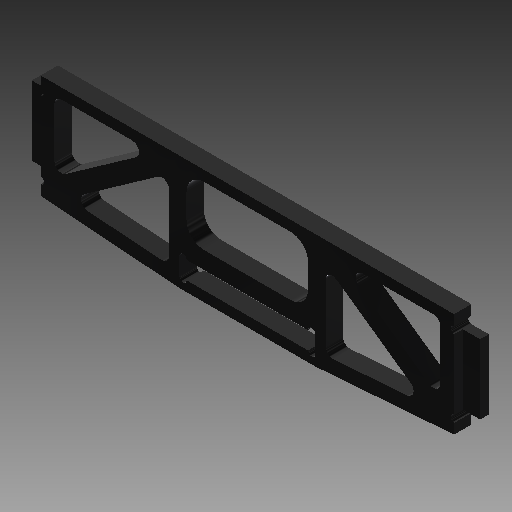
# Autodesk Inventor part: コックピット_サブフレーム_1_6
Saved by Autodesk Inventor 2018 (Build 220112000, 112)
## iProperties
Category: コックピット
Created: 2016-05-09
Part Number: コックピット_サブフレーム_1_6
Material: アセタール樹脂、黒
Document SubType Name: Modeling
Designer: hiroaki
Density: 1.425 g/cm^3
Appearance: 滑らか - 黒
Mass: 13.7144 g
Surface Area: 80.4855 cm^2
Volume: 9.62414 cm^3
Author: hiroaki
Autodesk Inventor part; units mm, degrees
ref_plane "YZ Plane" through (0, 0, 0) normal (1, 0, 0) x (0, 1, 0)
ref_plane "XZ Plane" through (0, 0, 0) normal (0, 1, 0) x (-1, 0, 0)
ref_plane "XY Plane" through (0, 0, 0) normal (0, 0, 1) x (1, 0, 0)
sketch "スケッチ1" plane through (0, 0, 0) normal (0, 0, 1) x (1, 0, 0)
  line L0 (-59.5, -15) -> (59.5, -15) construction
  line L1 (59.5, -15) -> (59.5, 15) construction
  line L2 (59.5, 15) -> (-59.5, 15) construction
  line L3 (-59.5, 15) -> (-59.5, -15) construction
  line L4 (-59.5, -15) -> (59.5, 15) construction
  line L5 (59.5, -15) -> (-59.5, 15) construction
  line L6 (-59.5, 12.1) -> (-59.5, 15)
  line L7 (-59.5, 15) -> (59.5, 15)
  line L8 (59.5, 15) -> (59.5, 12.1)
  line L9 (-59.5, -12.1) -> (-59.5, -15)
  line L10 (59.5, -15) -> (59.5, -12.1)
  line L11 (-59.5, 10) -> (-64.5, 10)
  line L12 (-64.5, 10) -> (-64.5, -10)
  line L13 (-64.5, -10) -> (-59.5, -10)
  arc A0 (-59.5, 10) -> (-59.5, 12.1) centre (-59.5, 11.05) ccw
  line L14 (0, 0) -> (0, 15) construction
  line L15 (0, 0) -> (-59.5, 0) construction
  arc A1 (-59.5, -12.1) -> (-59.5, -10) centre (-59.5, -11.05) ccw
  line L16 (59.5, 10) -> (64.5, 10)
  line L17 (64.5, 10) -> (64.5, -10)
  line L18 (64.5, -10) -> (59.5, -10)
  arc A2 (59.5, 12.1) -> (59.5, 10) centre (59.5, 11.05) ccw
  arc A3 (59.5, -10) -> (59.5, -12.1) centre (59.5, -11.05) ccw
  line L19 (-59.5, -15) -> (-19.5, -18)
  line L20 (-19.5, -18) -> (19.5, -18)
  line L21 (19.5, -18) -> (59.5, -15)
  line L22 (-19.5, -10) -> (19.5, -10) construction
  line L23 (19.5, -10) -> (19.5, -15) construction
  line L24 (19.5, -15) -> (-19.5, -15) construction
  line L25 (-19.5, -15) -> (-19.5, -10) construction
  line L26 (19.55, -9.95) -> (-19.55, -9.95)
  line L27 (-19.55, -9.95) -> (-19.55, -15.05)
  line L28 (-19.55, -15.05) -> (19.55, -15.05)
  line L29 (19.55, -15.05) -> (19.55, -9.95)
  circle A4 centre (-18.5, -9.95) radius 1.05
  circle A5 centre (-18.5, -15.05) radius 1.05
  circle A6 centre (18.5, -9.95) radius 1.05
  circle A7 centre (18.5, -15.05) radius 1.05
  dimension "d9" = 2.1
  dimension "d0" = 119
  dimension "d1" = 30
  dimension "d2" = 1.05
  dimension "d3" = 20
  dimension "d4" = 5
  dimension "d5" = 5
  dimension "d6" = 0.05
  dimension "d7" = 39
  dimension "d8" = 3
  constraints: 60 end point, 9 perpendicular, 8 point on circle, 6 collinear, 6 parallel, 6 vertical alignment, 5 horizontal, 4 centre point, 4 horizontal alignment, 4 midpoint, 4 point on line, 4 tangent, 3 equal radius, 2 symmetric about line, 2 vertical, 15 other
  measures "d0" distance of L1.end L2.end
  measures "d1" distance of L0.end L1.end
  measures "d2" radius of A0
  measures "d3" distance of L11.end L12.end
  measures "d4" distance between parallel lines of L3 L12
  measures "d5" distance of L24.end L22.start
  measures "d6" distance between parallel lines of L26 L22
  measures "d7" distance of L22.start L22.end
  measures "d8" distance between parallel lines of L20 L0
extrude "押し出し1" add sketch "スケッチ1" along normal blind 5
sketch "スケッチ2" plane through (0, 0, 5) normal (0, 0, 1) x (1, 0, 0)
  line L0 (59.5, 12.1) -> (59.5, 15) projected
  line L1 (-59.5, 15) -> (-59.5, 12.1) projected
  line L2 (65.6261, 13.972) -> (59.5, 13.972)
  line L3 (59.5, 13.972) -> (59.5, -16.1)
  line L4 (59.5, -16.1) -> (65.6261, -16.1)
  line L5 (65.6261, -16.1) -> (65.6261, 13.972)
  line L6 (-65.8886, -16.1) -> (-59.5, -16.1)
  line L7 (-59.5, -16.1) -> (-59.5, 18.3327)
  line L8 (-59.5, 18.3327) -> (-65.8886, 18.3327)
  line L9 (-65.8886, 18.3327) -> (-65.8886, -16.1)
  point P0 (0, 0)
  constraints: 16 end point, 4 parallel, 2 collinear, 2 horizontal, 2 perpendicular, 1 point on line
extrude "押し出し2" cut sketch "スケッチ2" against normal blind 2.5
sketch "スケッチ8" plane through (0, 0, 5) normal (0, 0, 1) x (1, 0, 0)
  line L0 (59.5, 15) -> (-59.5, 15) projected
  line L1 (-59.5, 10) -> (-59.5, -10) projected
  line L2 (-59.5, -15) -> (-19.5, -18) projected
  line L3 (17.45, -15.05) -> (-17.45, -15.05) projected
  arc A0 (-19.55, -15.05) -> (-17.45, -15.05) centre (-18.5, -15.05) ccw projected
  line L4 (-19.55, -15.05) -> (-19.55, -9.95) projected
  arc A1 (-17.45, -9.95) -> (-19.55, -9.95) centre (-18.5, -9.95) ccw projected
  line L5 (-17.45, -9.95) -> (17.45, -9.95) projected
  arc A2 (19.55, -9.95) -> (17.45, -9.95) centre (18.5, -9.95) ccw projected
  line L6 (19.55, -9.95) -> (19.55, -15.05) projected
  arc A3 (17.45, -15.05) -> (19.55, -15.05) centre (18.5, -15.05) ccw projected
  line L7 (-55.5, 12) -> (-22.5, 12) construction
  line L8 (-22.5, 12) -> (-22.5, -13.7638) construction
  line L9 (-22.5, -13.7638) -> (-55.5, -11.2888) construction
  line L10 (-55.5, -11.2888) -> (-55.5, 12) construction
  line L11 (17.5013, -10) -> (-17.5013, -10) construction
  arc A4 (-17.5013, -10) -> (-19.5, -9.95) centre (-18.5, -9.95) ccw construction
  line L12 (-19.5, -9.95) -> (-19.5, -15.05) construction
  arc A5 (-19.5, -15.05) -> (-17.5013, -15) centre (-18.5, -15.05) ccw construction
  line L13 (-17.5013, -15) -> (17.5013, -15) construction
  arc A6 (17.5013, -15) -> (19.5, -15.05) centre (18.5, -15.05) ccw construction
  line L14 (19.5, -15.05) -> (19.5, -9.95) construction
  arc A7 (19.5, -9.95) -> (17.5013, -10) centre (18.5, -9.95) ccw construction
  line L15 (-17.5, 12) -> (17.5, 12)
  line L16 (17.5, 12) -> (17.5, -5)
  line L17 (17.5, -5) -> (-17.5, -5)
  line L18 (-17.5, -5) -> (-17.5, 12)
  line L19 (0, 0) -> (0, 15) construction
  line L20 (-22.5, 12) -> (-55.5, -11.2888) construction
  line L21 (-55.5, 12) -> (-26.8358, 12)
  line L22 (-26.8358, 12) -> (-55.5, -8.2289)
  line L23 (-55.5, -8.2289) -> (-55.5, 12)
  line L24 (-51.5807, -11.5827) -> (-22.5, -13.7638)
  line L25 (-22.5, -13.7638) -> (-22.5, 8.9401)
  line L26 (-22.5, 8.9401) -> (-51.5807, -11.5827)
  line L27 (55.5, 12) -> (22.5, 12) construction
  line L28 (22.5, 12) -> (22.5, -13.7638) construction
  line L29 (22.5, -13.7638) -> (55.5, -11.2888) construction
  line L30 (55.5, -11.2888) -> (55.5, 12) construction
  line L31 (22.5, 12) -> (55.5, -11.2888) construction
  line L32 (55.5, 12) -> (26.8358, 12)
  line L33 (26.8358, 12) -> (55.5, -8.2289)
  line L34 (55.5, -8.2289) -> (55.5, 12)
  line L35 (51.5807, -11.5827) -> (22.5, -13.7638)
  line L36 (22.5, -13.7638) -> (22.5, 8.9401)
  line L37 (22.5, 8.9401) -> (51.5807, -11.5827)
  dimension "d51" = 4
  dimension "d52" = 3
  dimension "d53" = 0.05
  dimension "d54" = 3
  dimension "d55" = 4
  dimension "d56" = 5
  dimension "d57" = 5
  dimension "d58" = 5
  constraints: 62 end point, 10 symmetric about line, 8 point on circle, 6 parallel, 4 centre point, 4 collinear, 4 perpendicular, 3 horizontal, 1 horizontal alignment, 1 midpoint, 9 other
  measures "d51" distance between parallel lines of L10 L1
  measures "d52" distance between parallel lines of L0 L7
  measures "d53" distance between parallel lines of L5 L11
  measures "d54" distance between parallel lines of L12 L8
  measures "d55" distance between parallel lines of L2 L9
  measures "d56" distance between parallel lines of L11 L17
  measures "d57" distance between parallel lines of L18 L8
  measures "d58" distance between parallel lines of L26 L22
extrude "押し出し6" cut sketch "スケッチ8" against normal blind 10 contours L15 L16 L17 L18 | L21 L22 L23 | L26 L25 L24 | L34 L33 L32 | L35 L36 L37
fillet "フィレット4" radius 2 12 edges at (-55.5, 12, 2.5) (-55.5, -8.2289, 2.5) (-26.8358, 12, 2.5) (-22.5, 8.9401, 2.5) (-51.5807, -11.5827, 2.5) (-22.5, -13.7638, 2.5) (22.5, 8.9401, 2.5) (26.8358, 12, 2.5) (55.5, -8.2289, 2.5) (55.5, 12, 2.5) (22.5, -13.7638, 2.5) (51.5807, -11.5827, 2.5)
fillet "フィレット4" radius 5 4 edges at (-17.5, -5, 2.5) (-17.5, 12, 2.5) (17.5, 12, 2.5) (17.5, -5, 2.5)
